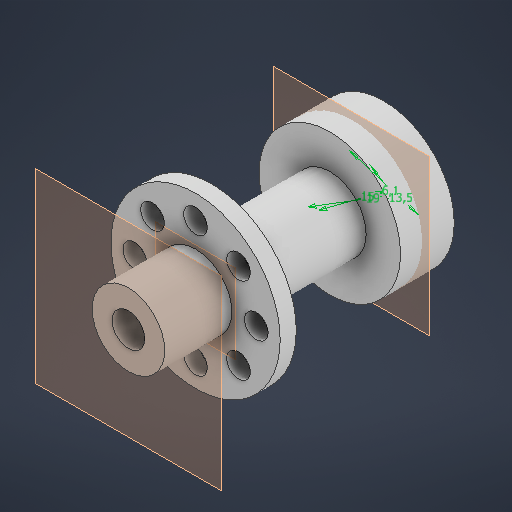
# Autodesk Inventor part: Затычка для Косозубки
Saved by Autodesk Inventor 2025 (Build 290162000, 162)
## iProperties
Created: 2025-09-25
Part Number: Затычка для Косозубки
Material: Типовые
Document SubType Name: Modeling
Designer: Phantom
Density: 1 g/cm^3
Appearance: По умолчанию
Author: Phantom
Autodesk Inventor part; units mm, degrees
ref_plane "YZ Plane" through (0, 0, 0) normal (1, 0, 0) x (0, 1, 0)
sketch "Эскиз1" plane through (0, 0, 0) normal (0, 0, 1) x (1, 0, 0)
  circle A0 centre (0, 0) radius 6.75
  circle A1 centre (0, 0) radius 3.05
  dimension "d0" = 13.5
  dimension "d1" = 6.1
  constraints: 2 centre point, 2 coincident
  measures "d0" diameter of A0
  measures "d1" diameter of A1
ref_plane "РабПлоскость1" through (0, 0, 35) normal (0, 0, 1) x (1, 0, 0)
sketch "Эскиз2" plane through (0, 0, 35) normal (0, 0, 1) x (1, 0, 0)
  circle A0 centre (0, 0) radius 15.75
  dimension "d5" = 31.5
  constraints: 1 centre point, 1 coincident
  measures "d5" diameter of A0
extrude "Выдавливание2" add sketch "Эскиз2" against normal blind 3
sketch "Эскиз3" plane through (0, 0, 35) normal (0, 0, 1) x (1, 0, 0)
  line L0 (0, 0) -> (0, 11.319)
  line L1 (0, 0) -> (11.319, 0) construction
  circle A0 centre (0, 11.319) radius 2.2
  circle A1 centre (0, 0) radius 1.4142
  circle A2 centre (-8.0037, 8.0037) radius 2.2
  circle A3 centre (-11.319, 0) radius 2.2
  circle A4 centre (-8.0037, -8.0037) radius 2.2
  circle A5 centre (0, -11.319) radius 2.2
  circle A6 centre (8.0037, -8.0037) radius 2.2
  circle A7 centre (11.319, 0) radius 2.2
  circle A8 centre (8.0037, 8.0037) radius 2.2
  dimension "d8" = 11.319
  dimension "d9" = 90
  dimension "d10" = 4.4
  dimension "d13" = 360
  constraints: 9 centre point, 4 end point, 2 coincident, 1 horizontal, 1 perpendicular, 1 vertical, 17 other
  measures "d8" distance of L0.start L0.end
  measures "d9" angle of L1 L0
  measures "d10" diameter of A0
extrude "Выдавливание3" cut sketch "Эскиз3" against normal blind 3 contours A0 | A2 | A3 | A4 | A5 | A6 | A7 | A8
ref_plane "РабПлоскость4" through (0, 0, 0) normal (0, 0, -1) x (-1, 0, 0)
sketch "Эскиз4" plane through (0, 0, 0) normal (0, 0, -1) x (-1, 0, 0)
  circle A0 centre (0, 0) radius 13.15
  circle A1 centre (0, 0) radius 9.5
  dimension "d17" = 26.3
  dimension "d18" = 19
  constraints: 2 centre point, 2 coincident
  measures "d17" diameter of A0
  measures "d18" diameter of A1
extrude "Выдавливание4" add sketch "Эскиз4" against normal blind 10
ref_plane "РабПлоскость2" through (0, 0, 7) normal (0, 0, 1) x (1, 0, 0)
ref_plane "РабПлоскость3" through (0, 0, 47.5) normal (0, 0, 1) x (1, 0, 0)
sketch "Эскиз6" plane through (0, 0, 47.5) normal (0, 0, 1) x (1, 0, 0)
  circle A0 centre (0, 0) radius 6.75
  circle A1 centre (0, 0) radius 3.05
  dimension "d28" = 13.5
  dimension "d29" = 6.1
  constraints: 2 centre point, 2 coincident
  measures "d28" diameter of A0
  measures "d29" diameter of A1
ref_plane "РабПлоскость5" through (0, 0, 6) normal (0, 0, 1) x (1, 0, 0)
sketch "Эскиз7" plane through (0, 0, 6) normal (0, 0, 1) x (1, 0, 0)
  circle A0 centre (0, 0) radius 7.5
  circle A1 centre (0, 0) radius 9.5
  dimension "d31" = 15
  dimension "d32" = 19
  constraints: 2 centre point, 2 coincident
  measures "d31" diameter of A0
  measures "d32" diameter of A1
extrude "Выдавливание7" add sketch "Эскиз7" along normal blind 4 contours A0 | A1
extrude "Выдавливание8" cut sketch "Эскиз7" along normal blind 1 contours A0
extrude "Выдавливание9" add sketch "Эскиз6" against normal blind 38.5
